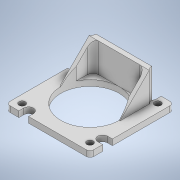
# Autodesk Inventor part: MotorCrepper2
Saved by Autodesk Inventor 2020.1 (Build 241239000, 239)
## iProperties
Created: 2023-01-14
Part Number: MotorCrepper2
Material: Типовые
Document SubType Name: Modeling
Designer: KirikDK
Density: 1 g/cm^3
Appearance: По умолчанию
Author: KirikDK
Autodesk Inventor part; units mm, degrees
ref_plane "YZ Plane" through (0, 0, 0) normal (1, 0, 0) x (0, 1, 0)
ref_plane "XZ Plane" through (0, 0, 0) normal (0, 1, 0) x (-1, 0, 0)
ref_plane "XY Plane" through (0, 0, 0) normal (0, 0, 1) x (1, 0, 0)
sketch "Эскиз1" plane through (0, 0, 0) normal (0, 1, 0) x (-1, 0, 0)
  arc A0 (82, -4) -> (78, 0) centre (78, -4) ccw
  line L0 (82, -63) -> (82, -4)
  line L1 (-4, -23) -> (-4, -82)
  line L2 (1, -23) -> (-4, -23)
  arc A1 (1, -23) -> (6, -18) centre (1, -18) ccw
  arc A2 (6, -18) -> (1, -13) centre (1, -18) ccw
  circle A3 centre (39, -43) radius 30
  line L3 (-4, -13) -> (1, -13)
  line L4 (-4, -4) -> (-4, -13)
  arc A4 (0, 0) -> (-4, -4) centre (0, -4) ccw
  line L5 (59, 0) -> (0, 0)
  line L6 (59, -5) -> (59, 0)
  line L7 (78, 0) -> (69, 0)
  arc A5 (59, -5) -> (69, -5) centre (64, -5) ccw
  line L8 (69, 0) -> (69, -5)
  arc A6 (77.1, -8.2) -> (70.5, -8.2) centre (73.8, -8.2) ccw
  circle A7 centre (73.8, -8.2) radius 3.3
  circle A8 centre (4.2, -8.2) radius 3.3
  circle A9 centre (73.8, -77.8) radius 3.3
  circle A10 centre (4.2, -77.8) radius 3.3
  arc A11 (19, -81) -> (9, -81) centre (14, -81) ccw
  line L9 (19, -81) -> (19, -86)
  line L10 (9, -86) -> (9, -81)
  line L11 (0, -86) -> (9, -86)
  arc A12 (-4, -82) -> (0, -86) centre (0, -82) ccw
  line L12 (19, -86) -> (78, -86)
  arc A13 (78, -86) -> (82, -82) centre (78, -82) ccw
  line L13 (82, -82) -> (82, -73)
  line L14 (82, -73) -> (77, -73)
  arc A14 (77, -63) -> (77, -73) centre (77, -68) ccw
  line L15 (77, -63) -> (82, -63)
  point P0 (0, 0)
  constraints: 32 end point, 20 point on circle, 15 centre point
extrude "Выдавливание1" add sketch "Эскиз1" along normal blind 6
sketch "Эскиз2" plane through (0, 6, 0) normal (0, 1, 0) x (1, 0, 0)
  line L0 (4, 23) -> (4, 82) projected
  line L1 (-82, 85.8) -> (4, 85.8)
  line L2 (4, 85.8) -> (4, 77.8)
  line L3 (4, 77.8) -> (-82, 77.8)
  line L4 (-82, 77.8) -> (-82, 85.8)
  circle A0 centre (-73.8, 77.8) radius 3.3 projected
  circle A1 centre (-4.2, 77.8) radius 3.3 projected
  circle A2 centre (-4.2, 77.8) radius 6.2032
  circle A3 centre (-73.8, 77.8) radius 6.2032
  line L5 (-82, 73) -> (-77, 73) projected
  line L6 (-82, 73) -> (4, 73)
  line L7 (4, 73) -> (4, 77.8)
  line L8 (4, 77.8) -> (-82, 77.8)
  line L9 (-82, 77.8) -> (-82, 73)
  line L10 (-8.1294, 73) -> (-12, 73)
  line L11 (-12, 73) -> (-12, 42.9076)
  line L12 (-12, 42.9076) -> (-8.1294, 42.9076)
  line L13 (-8.1294, 42.9076) -> (-8.1294, 73)
  line L14 (-69.8706, 73) -> (-66.037, 73)
  line L15 (-66.037, 73) -> (-66.037, 42.9076)
  line L16 (-66.037, 42.9076) -> (-69.8706, 42.9076)
  line L17 (-69.8706, 42.9076) -> (-69.8706, 73)
  circle A4 centre (-39, 43) radius 30 projected
  point P0 (0, 0)
  point P1 (-80.0032, 77.8)
  point P2 (-67.5968, 77.8)
  point P3 (-10.4032, 77.8)
  point P4 (2.0032, 77.8)
  point P5 (-12, 56.0767)
  point P6 (-9.0001, 42.9076)
  point P7 (-68.9999, 42.9076)
  point P8 (-66.037, 56)
  dimension "d4" = 4.8
  dimension "d5" = 8
  constraints: 32 end point, 8 parallel, 5 point on line, 4 horizontal, 4 perpendicular, 2 coincident, 6 other
  measures "d4" distance of L8.end L5.start
  measures "d5" distance of L3.end L1.start
extrude "Выдавливание3" add sketch "Эскиз2" along normal blind 30 contours L6 A3 L3 A2 | L13 L12 A4 L11 L6 | L6 L15 A4 L16 L17
chamfer "Фаска1" distance 30 angle 45 2 edges at (-69.4352, 36, -42.9076) (-8.5648, 36, -42.9076)
fillet "Сопряжение1" radius 6 2 edges at (-66.037, 21, -73) (-12, 21, -73)
